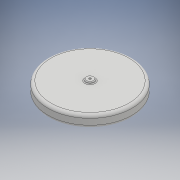
# Autodesk Inventor part: 前輪
Saved by Autodesk Inventor 2018 (Build 220112000, 112)
## iProperties
Created: 2017-09-09
Part Number: 前輪
Material: 一般
Document SubType Name: Modeling
Designer: Kenta
Density: 1 g/cm^3
Appearance: 既定
Author: Kenta
Autodesk Inventor part; units mm, degrees
ref_plane "YZ Plane" through (0, 0, 0) normal (1, 0, 0) x (0, 1, 0)
ref_plane "XZ Plane" through (0, 0, 0) normal (0, 1, 0) x (-1, 0, 0)
ref_plane "XY Plane" through (0, 0, 0) normal (0, 0, 1) x (1, 0, 0)
sketch "スケッチ1" plane through (0, 0, 0) normal (0, 0, 1) x (1, 0, 0)
  circle A0 centre (0, 0) radius 245
  dimension "d0" = 490
  constraints: 1 centre point, 1 coincident
  measures "d0" diameter of A0
extrude "押し出し1" add sketch "スケッチ1" along normal mid plane 70
fillet "フィレット1" radius 17.5 2 edges at (-245, 0, 35) (-245, 0, -35)
sketch "スケッチ8" plane through (0, 0, 35) normal (0, 0, 1) x (1, 0, 0)
  circle A0 centre (0, 0) radius 25
  dimension "d11" = 50
  constraints: 1 centre point, 1 coincident
  measures "d11" diameter of A0
extrude "押し出し2" add sketch "スケッチ8" along normal blind 10
sketch "スケッチ9" plane through (0, 0, -35) normal (0, 0, -1) x (-1, 0, 0)
  circle A0 centre (0, 0) radius 120
  dimension "d14" = 240
  constraints: 1 centre point, 1 coincident
  measures "d14" diameter of A0
extrude "押し出し3" add sketch "スケッチ9" along normal blind 35
fillet "フィレット2" radius 5 1 edges at (-25, 0, 45)
fillet "フィレット3" radius 5 1 edges at (-25, 0, 35)
fillet "フィレット4" radius 5 2 edges at (120, 0, -70) (120, 0, -35)
sketch "スケッチ10" plane through (0, 0, -70) normal (0, 0, -1) x (-1, 0, 0)
  point P0 (0, 0)
  point P1 (0, 0)
  constraints: 1 coincident
hole "穴2" at (0, 0, -70) direction (0, 0, 1) diameter 12 end through all
